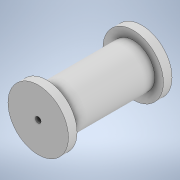
# Autodesk Inventor part: DrumM8
Saved by Autodesk Inventor 2020 (Build 240168000, 168)
## iProperties
Created: 2020-06-05
Part Number: DrumM8
Material: Generic
Document SubType Name: Modeling
Designer: jurre
Density: 1 g/cm^3
Appearance: Default
Author: jurre
Autodesk Inventor part; units mm, degrees
ref_plane "YZ Plane" through (0, 0, 0) normal (1, 0, 0) x (0, 1, 0)
ref_plane "XZ Plane" through (0, 0, 0) normal (0, 1, 0) x (-1, 0, 0)
ref_plane "XY Plane" through (0, 0, 0) normal (0, 0, 1) x (1, 0, 0)
sketch "Sketch1" plane through (0, 0, 0) normal (0, 0, 1) x (1, 0, 0)
  circle A0 centre (0, 0) radius 35
  dimension "d0" = 70
  constraints: 1 centre point, 1 coincident
  measures "d0" diameter of A0
extrude "Extrusion1" add sketch "Sketch1" along normal blind 10
sketch "Sketch2" plane through (0, 0, 0) normal (0, 0, -1) x (-1, 0, 0)
  line L0 (0, -8.0829) -> (-7, -4.0415)
  line L1 (-7, -4.0415) -> (-7, 4.0415)
  line L2 (-7, 4.0415) -> (0, 8.0829)
  line L3 (0, 8.0829) -> (7, 4.0415)
  line L4 (7, 4.0415) -> (7, -4.0415)
  line L5 (7, -4.0415) -> (0, -8.0829)
  point P0 (0, 0)
  point P1 (0, 0)
  dimension "d3" = 14
  constraints: 12 end point, 1 coincident, 13 other
  measures "d3" distance between parallel lines of L4 L1
extrude "Extrusion2" cut sketch "Sketch2" against normal blind 7
sketch "Sketch3" plane through (0, 0, 7) normal (0, 0, -1) x (-1, 0, 0)
  point P0 (0, 0)
sketch "Sketch4" plane through (0, 0, 10) normal (0, 0, 1) x (1, 0, 0)
  circle A0 centre (0, 0) radius 25
  dimension "d6" = 50
  constraints: 1 centre point, 1 coincident
  measures "d6" diameter of A0
extrude "Extrusion3" add sketch "Sketch4" along normal blind 100
sketch "Sketch5" plane through (0, 0, 110) normal (0, 0, 1) x (1, 0, 0)
  circle A0 centre (0, 0) radius 35
  constraints: 1 centre point, 1 coincident
extrude "Extrusion4" add sketch "Sketch5" along normal blind 10
hole "Hole1" at (0, 0, 7) direction (0, 0, 1) diameter 6.647 end through all thread size "M8x1.25" class "6H" standard "ISO Metric profile"
body "Solid1"
